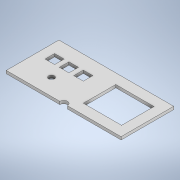
# Autodesk Inventor part: Circuit Cover
Saved by Autodesk Inventor 2022 (Build 260153000, 153)
## iProperties
Created: 2022-05-06
Part Number: Circuit Cover
Material: Generic
Document SubType Name: Modeling
Designer: Jeanette Guo
Density: 1 g/cm^3
Appearance: Default
Author: Jeanette Guo
Autodesk Inventor part; units mm, degrees
ref_plane "YZ Plane" through (0, 0, 0) normal (1, 0, 0) x (0, 1, 0)
ref_plane "XZ Plane" through (0, 0, 0) normal (0, 1, 0) x (-1, 0, 0)
ref_plane "XY Plane" through (0, 0, 0) normal (0, 0, 1) x (1, 0, 0)
sketch "Sketch1" plane through (0, 0, 0) normal (0, 1, 0) x (-1, 0, 0)
  line L0 (5, -4.9911) -> (15, -4.9911)
  line L1 (15, -4.9911) -> (15, -14.9911)
  line L2 (15, -14.9911) -> (5, -14.9911)
  line L3 (5, -14.9911) -> (5, -4.9911)
  line L4 (5, -4.9911) -> (15, -14.9911) construction
  line L5 (15, -4.9911) -> (5, -14.9911) construction
  line L6 (20, -4.9911) -> (30, -4.9911)
  line L7 (30, -4.9911) -> (30, -14.9911)
  line L8 (30, -14.9911) -> (20, -14.9911)
  line L9 (20, -14.9911) -> (20, -4.9911)
  line L10 (20, -4.9911) -> (30, -14.9911) construction
  line L11 (30, -4.9911) -> (20, -14.9911) construction
  line L12 (35, -4.9911) -> (45, -4.9911)
  line L13 (45, -4.9911) -> (45, -14.9911)
  line L14 (45, -14.9911) -> (35, -14.9911)
  line L15 (35, -14.9911) -> (35, -4.9911)
  line L16 (35, -4.9911) -> (45, -14.9911) construction
  line L17 (45, -4.9911) -> (35, -14.9911) construction
  circle A0 centre (25, 8.2297) radius 3
  line L18 (-55, 15.0089) -> (-15, 15.0089)
  line L19 (-15, 15.0089) -> (-15, -18.9911)
  line L20 (-15, -18.9911) -> (-55, -18.9911)
  line L21 (-55, -18.9911) -> (-55, 15.0089)
  line L22 (-58, -24.9656) -> (-58, -25)
  line L23 (58, -29.4911) -> (58, 25.5089)
  line L24 (-68, 25.5089) -> (-68, -29.4911)
  line L25 (-68, 22.0706) -> (-55, 22.0706)
  line L26 (-68, 25.5089) -> (58, 25.5089)
  line L27 (58, 17.0063) -> (45, 17.0063)
  line L28 (-68, -29.4911) -> (-50, -29.4911)
  line L29 (-50, -29.4911) -> (-50, -32.4911)
  line L30 (-50, -32.4911) -> (40, -32.4911)
  line L31 (40, -32.4911) -> (40, -29.4911)
  line L32 (40, -29.4911) -> (58, -29.4911)
  line L33 (-68, 22.0706) -> (-65, 22.0706)
  line L34 (-65, 17.0063) -> (-65, -29.4911)
  line L35 (58, -29.4911) -> (55, -29.4911)
  line L36 (55, -29.4911) -> (55, 25.5089)
  line L37 (-65, 17.0063) -> (-65, 25.5089)
  line L38 (40, -29.4911) -> (-50, -29.4911)
  arc A1 (-9, 25.5089) -> (-1, 25.5089) centre (-5, 25.5089) ccw
  point P0 (0, 0)
  point P1 (10, -9.9911)
  point P2 (25, -9.9911)
  point P3 (40, -9.9911)
  point P4 (-23.3045, 0)
  point P5 (-35, -18.9911)
  point P6 (-35, -20.979)
  point P7 (-55, -25)
  point P8 (-58, -29.4911)
  point P9 (25, -4.9911)
  point P10 (10, -9.9911)
  point P11 (25, -9.9911)
  point P12 (25, -9.9911)
  point P13 (40, -9.9911)
  dimension "d11" = 10
  dimension "d12" = 10
  dimension "d13" = 10
  dimension "d14" = 10
  dimension "d15" = 10
  dimension "d16" = 10
  dimension "d17" = 5
  dimension "d18" = 5
  dimension "d20" = 6
  dimension "d21" = 40
  dimension "d22" = 34
  dimension "d81" = 126
  dimension "d83" = 13
  dimension "d84" = 18
  dimension "d85" = 90
  dimension "d87" = 3
  dimension "d88" = 13
  dimension "d90" = 4
  dimension "d91" = 10.5
  dimension "d93" = 55
  dimension "d94" = 10.5
  dimension "d95" = 14.5
  dimension "d98" = 18.2208
  constraints: 78 end point, 13 midpoint, 11 point on line, 10 perpendicular, 9 horizontal, 9 parallel, 4 vertical alignment, 2 centre point, 2 horizontal alignment, 2 point on circle
  measures "d11" distance of L1.end L2.end
  measures "d12" distance of L0.end L1.end
  measures "d13" distance of L7.end L8.end
  measures "d14" distance of L6.end L7.end
  measures "d15" distance of L13.end L14.end
  measures "d16" distance of L12.end L13.end
  measures "d17" distance between parallel lines of L9 L1
  measures "d18" distance between parallel lines of L15 L7
  measures "d20" diameter of A0
  measures "d21" distance of L19.end L20.end
  measures "d22" distance of L18.end L19.end
  measures "d81" distance of L24.start L23.end
  measures "d83" distance of L27.start L27.end
  measures "d84" distance of L24.end L28.end
  measures "d85" distance of L29.end L30.end
  measures "d87" distance of L23.start L35.end
  measures "d88" distance of L25.start L25.end
  measures "d90" radius of A1
  measures "d91" distance between parallel lines of L20 L38
  measures "d93" distance of L24.start L24.end
  measures "d94" distance between parallel lines of L26 L18
  measures "d95" distance between parallel lines of L8 L38
  measures "d98" distance of A0.centre point (25, -9.991)
extrude "Extrusion1" add sketch "Sketch1" along normal blind 3 contours L32 L38 L28 L34 L37 L26 A1 L36
body "Solid1"
